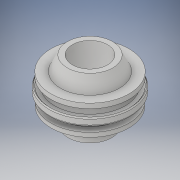
# Autodesk Inventor part: Section Adaptor WIP
Saved by Autodesk Inventor 2017 (Build 210142000, 142)
## iProperties
Created: 2016-11-04
Part Number: Section Adaptor WIP
Material: Generic
Document SubType Name: Modeling
Designer: lieub
Density: 1 g/cm^3
Appearance: Default
Author: lieub
Autodesk Inventor part; units mm, degrees
ref_plane "YZ Plane" through (0, 0, 0) normal (1, 0, 0) x (0, 1, 0)
ref_plane "XZ Plane" through (0, 0, 0) normal (0, 1, 0) x (-1, 0, 0)
ref_plane "XY Plane" through (0, 0, 0) normal (0, 0, 1) x (1, 0, 0)
sketch "Sketch1" plane through (0, 0, 0) normal (0, 0, 1) x (1, 0, 0)
  line L0 (0, 0) -> (0, 25.4713) construction
  line L1 (-206.1253, 8.0706) -> (-206.1253, -17.3294)
  line L2 (-206.1253, -17.3294) -> (-203.2, -23.287)
  line L3 (-203.2, -23.287) -> (-203.2, -17.3294)
  line L4 (-203.2, -17.3294) -> (-196.85, -17.3294)
  line L5 (-196.85, -17.3294) -> (-196.85, -18.6213)
  line L6 (-206.1253, 8.0706) -> (-202.8327, 15.2137)
  line L7 (-202.8327, 15.2137) -> (-202.8327, 8.0706)
  line L8 (-202.8327, 8.0706) -> (-196.8015, 8.0706)
  line L9 (-196.8015, 8.0706) -> (-196.8015, 9.3626)
  line L10 (-196.8015, 9.3626) -> (-177.369, 9.3626)
  line L11 (-196.85, -18.6213) -> (-177.4174, -18.6213)
  line L12 (-159.6027, 47.4626) -> (-196.85, 47.4626)
  line L13 (-196.85, 47.4626) -> (-196.85, 71.7094)
  line L14 (-196.85, 71.7094) -> (-148.2962, 71.7094)
  line L15 (-159.6511, -56.7213) -> (-195.9938, -56.7213)
  line L16 (-195.9938, -56.7213) -> (-195.9938, -78.0553)
  line L17 (-195.9938, -78.0553) -> (-149.7029, -78.0553)
  line L18 (-177.369, 9.3626) -> (-159.6027, 47.4626)
  line L19 (-148.2962, 71.7094) -> (-143.6137, 81.751)
  line L20 (-177.4174, -18.6213) -> (-159.6511, -56.7213)
  line L21 (-149.7029, -78.0553) -> (-143.013, -92.4018)
  line L22 (-143.6137, 81.751) -> (-114.6581, 143.8464)
  line L23 (-143.013, -92.4018) -> (-109.7002, -163.8414)
  line L24 (-114.6581, 143.8464) -> (-88.6327, 143.8464)
  line L25 (-88.6327, 143.8464) -> (-88.6327, -163.8414)
  line L26 (-88.6327, -163.8414) -> (-109.7002, -163.8414)
  dimension "d0" = 6.35
  dimension "d3" = 203.2
  dimension "d11" = 38.1
  dimension "d12" = 38.1
  dimension "d13" = 0
  dimension "d14" = 25.4
  dimension "d15" = 0
  dimension "d16" = 115
  dimension "d17" = 115
  constraints: 54 end point, 9 perpendicular, 6 vertical, 4 horizontal, 2 parallel
  measures "d0" distance of L3.end L4.end
  measures "d3" distance from line of L0 L3.end
  measures "d11" vertical distance of L12.start L10.end
  measures "d12" vertical distance of L15.start L11.end
  measures "d13" distance from line of L1.start L8
  measures "d14" distance of L1.start L1.end
  measures "d15" distance from line of L1.end L4
  measures "d16" angle of L23 L17
  measures "d17" angle of L22 L14
revolve "Revolution1" add sketch "Sketch1" angle 360 about axis through (0, 0, 0) along (0, 1, 0)
body "Solid1"
